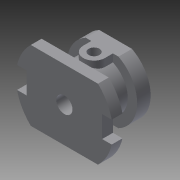
# Autodesk Inventor part: 零件7-20-2
Saved by Autodesk Inventor 2014 (Build 180170000, 170)
## iProperties
Created: 2018-12-21
Part Number: 零件7-20-2
Material: 常规
Document SubType Name: Modeling
Designer: Administrator
Density: 1 g/cm^3
Appearance: 默认
Author: Administrator
Autodesk Inventor part; units mm, degrees
ref_plane "YZ Plane" through (0, 0, 0) normal (1, 0, 0) x (0, 1, 0)
ref_plane "XZ Plane" through (0, 0, 0) normal (0, 1, 0) x (-1, 0, 0)
ref_plane "XY Plane" through (0, 0, 0) normal (0, 0, 1) x (1, 0, 0)
sketch "草图1" plane through (0, 0, 0) normal (0, 1, 0) x (-1, 0, 0)
  line L0 (12.4499, -13) -> (-12.4499, -13)
  line L1 (12.4499, 13) -> (-12.4499, 13)
  line L2 (21.8859, 0) -> (-29.1909, 0)
  line L3 (17.5499, 4) -> (14, 4)
  line L4 (14, 4) -> (14, -4)
  line L5 (14, -4) -> (17.5499, -4)
  line L6 (22, 4) -> (14, -4) construction
  line L7 (14, 4) -> (22, -4) construction
  line L8 (-17.5499, 4) -> (-14, 4)
  line L9 (-14, 4) -> (-14, -4)
  line L10 (-14, -4) -> (-17.5499, -4)
  line L11 (-22, 4) -> (-14, -4) construction
  line L12 (-14, 4) -> (-22, -4) construction
  arc A0 (12.4499, -13) -> (17.5499, -4) centre (0, 0) ccw
  arc A1 (17.5499, 4) -> (12.4499, 13) centre (0, 0) ccw
  arc A2 (-12.4499, 13) -> (-17.5499, 4) centre (0, 0) ccw
  arc A3 (-17.5499, -4) -> (-12.4499, -13) centre (0, 0) ccw
  point P0 (18, 0)
  point P1 (-18, 0)
  dimension "d1" = 26
  dimension "d2" = 8
  dimension "d3" = 8
  dimension "d4" = 8
  dimension "d5" = 8
  constraints: 26 end point, 10 point on circle, 4 centre point, 4 midpoint, 4 parallel, 3 horizontal, 2 perpendicular, 1 coincident, 1 point on line, 1 other
  measures "d1" distance between parallel lines of L1 L0
  measures "d2" distance of L7.end L4.end
  measures "d3" distance of L9.end L12.end
  measures "d4" distance of L3.end L4.end
  measures "d5" distance of L8.end L9.end
extrude "拉伸1" add sketch "草图1" along normal blind 4
sketch "草图2" plane through (0, 4, 0) normal (0, 1, 0) x (1, 0, 0)
  arc A0 (17.5499, 4) -> (12.4499, 13) centre (0, 0) ccw projected
  circle A1 centre (0, 0) radius 9.5
  dimension "d8" = 19
  constraints: 1 centre point, 1 coincident
  measures "d8" diameter of A1
extrude "拉伸2" add sketch "草图2" along normal blind 10
sketch "草图3" plane through (0, 14, 0) normal (0, 1, 0) x (1, 0, 0)
  circle A0 centre (0, 0) radius 9.5 projected
  circle A1 centre (0, 0) radius 13
  dimension "d11" = 26
  constraints: 1 centre point, 1 coincident
  measures "d11" diameter of A1
extrude "拉伸3" add sketch "草图3" along normal blind 5 contours A0 | A1
sketch "草图4" plane through (0, 19, 0) normal (0, 1, 0) x (1, 0, 0)
  circle A0 centre (0, 0) radius 13 projected
  line L0 (-22.4415, 0) -> (25.3714, 0)
  line L1 (-6.0622, 11.5) -> (6.0622, 11.5)
  line L2 (-6.0622, -11.5) -> (6.0622, -11.5)
  dimension "d14" = 23
  constraints: 6 end point, 4 point on circle, 2 parallel, 1 horizontal, 1 point on line, 1 other
  measures "d14" distance between parallel lines of L2 L1
extrude "拉伸4" cut sketch "草图4" against normal blind 5 contours L1 A0 | A0 L2
sketch "草图5" plane through (-6.0622, 19, 11.5) normal (0, 0, 1) x (1, 0, 0)
  line L0 (0, 0) -> (12.1244, 0) projected
  line L1 (15.5622, -5) -> (-3.4378, -5) projected
  line L2 (-3.4378, -15) -> (15.5622, -15) projected
  line L3 (6.0622, -19) -> (6.0622, 3.3866)
  line L4 (2.0622, -8) -> (2.0622, -5)
  line L5 (2.0622, -5) -> (10.0622, -5)
  line L6 (10.0622, -5) -> (10.0622, -8)
  line L7 (10.0622, -8) -> (2.0622, -5) construction
  line L8 (2.0622, -8) -> (10.0622, -5) construction
  arc A0 (2.0622, -8) -> (10.0622, -8) centre (6.0622, -8) ccw
  point P0 (6.0622, -6.5)
  dimension "d17" = 8
  dimension "d18" = 3
  constraints: 12 end point, 3 point on line, 2 midpoint, 2 point on circle, 1 centre point, 1 parallel, 1 perpendicular
  measures "d17" distance of L4.end L5.end
  measures "d18" distance of L6.end L5.end
extrude "拉伸5" add sketch "草图5" against normal blind 5
sketch "草图6" plane through (6.0622, 19, -11.5) normal (0, 0, -1) x (-1, 0, 0)
  line L0 (10.0622, -8) -> (10.0622, -5) projected
  line L1 (2.0622, -5) -> (10.0622, -5) projected
  line L2 (2.0622, -5) -> (2.0622, -8) projected
  line L3 (-3.4378, -15) -> (15.5622, -15) projected
  spline S0 degree 2 poles (2.0622, -8) (2.0622, -12) (6.0622, -12) (10.0622, -12) (10.0622, -8) knots 0 0 0 0.5 0.5 1 1 1 weights 1 0.707107 1 0.707107 1 projected
  point P0 (6.0622, -19)
  constraints: 2 horizontal alignment
extrude "拉伸6" add sketch "草图6" against normal blind 5
sketch "草图7" plane through (-6.0622, 19, 11.5) normal (0, 0, 1) x (1, 0, 0)
  arc A0 (2.0622, -8) -> (10.0622, -8) centre (6.0622, -8) ccw projected
  circle A1 centre (6.0622, -8) radius 2
  point P0 (6.0622, -19)
  dimension "d23" = 4
  constraints: 1 centre point, 1 coincident
  measures "d23" diameter of A1
extrude "拉伸7" cut sketch "草图7" against normal blind 30
sketch "草图8" plane through (0, 19, 0) normal (0, 1, 0) x (1, 0, 0)
  arc A0 (6.0622, -11.5) -> (6.0622, 11.5) centre (0, 0) ccw projected
  circle A1 centre (0, 0) radius 7
  dimension "d26" = 14
  constraints: 1 centre point, 1 coincident
  measures "d26" diameter of A1
extrude "拉伸8" cut sketch "草图8" against normal blind 13
sketch "草图9" plane through (0, 0, 0) normal (0, -1, 0) x (1, 0, 0)
  arc A0 (-17.5499, -4) -> (-12.4499, -13) centre (0, 0) ccw projected
  circle A1 centre (0, 0) radius 3
  dimension "d29" = 6
  constraints: 1 centre point, 1 coincident
  measures "d29" diameter of A1
extrude "拉伸9" cut sketch "草图9" against normal blind 13
